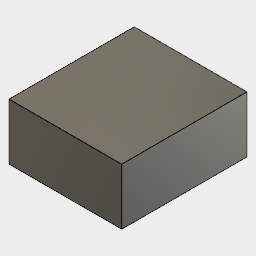
testFusion v1 (Autodesk Fusion 360 design; units mm, degrees)
Autodesk Fusion 360 part; units mm, degrees
sketch "Sketch1" plane through (0, 0, 0) normal (0, 0, 1) x (1, 0, 0)
  line L0 (-70, 20) -> (20, 20)
  line L1 (20, 20) -> (20, -25)
  line L2 (20, -25) -> (-70, -25)
  line L3 (-70, -25) -> (-70, 20)
  line L4 (-25, -5) -> (52.74, -5)
  line L5 (52.74, -5) -> (52.74, 65.0457)
  line L6 (52.74, 65.0457) -> (-25, 65.0457)
  line L7 (-25, 65.0457) -> (-25, -5)
  constraint horizontal L0
  constraint vertical L1
  constraint horizontal L2
  constraint vertical L3
  constraint horizontal L4
  constraint vertical L5
  constraint horizontal L6
  constraint vertical L7
extrude "Extrude1" add sketch "Sketch1" along normal blind 100 contours L0 L1 L2 L3 L4 L7 | L0 L1 L4 L7
